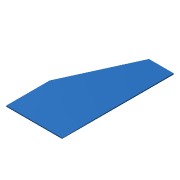
# Autodesk Inventor part: SidePanel
Saved by Autodesk Inventor 2014 (Build 180170000, 170)
## iProperties
Created: 2014-08-10
Part Number: SidePanel
Material: Generic
Document SubType Name: Modeling
Designer: Peele
Density: 1 g/cm^3
Appearance: Cyan
Author: Peele
Autodesk Inventor part; units mm, degrees
ref_plane "YZ Plane" through (0, 0, 0) normal (1, 0, 0) x (0, 1, 0)
ref_plane "XZ Plane" through (0, 0, 0) normal (0, 1, 0) x (-1, 0, 0)
ref_plane "XY Plane" through (0, 0, 0) normal (0, 0, 1) x (1, 0, 0)
sketch "Sketch1" plane through (0, 0, 0) normal (0, 0, 1) x (1, 0, 0)
  line L0 (-112.5, -225) -> (112.5, -225)
  line L1 (112.5, -225) -> (112.5, 225)
  line L2 (112.5, 225) -> (-112.5, 225)
  line L3 (-112.5, 225) -> (-112.5, -225)
  line L4 (-112.5, -225) -> (112.5, 225) construction
  line L5 (112.5, -225) -> (-112.5, 225) construction
  point P0 (0, 0)
  dimension "d0" = 225
  dimension "d1" = 450
  constraints: 12 end point, 2 midpoint, 2 parallel, 1 horizontal, 1 perpendicular
  measures "d0" distance of L1.end L2.end
  measures "d1" distance of L2.end L0.start
extrude "Extrusion1" add sketch "Sketch1" along normal blind 4
sketch "Sketch2" plane through (0, 0, 4) normal (0, 0, 1) x (1, 0, 0)
  line L0 (-112.5, 225) -> (12.5, 225)
  line L1 (12.5, 225) -> (-112.5, -50)
  line L2 (-112.5, 225) -> (-112.5, -50)
  line L3 (112.5, -225) -> (112.5, 225) projected
  line L4 (112.5, -50) -> (112.5, 225)
  line L5 (112.5, 225) -> (62.5, 225)
  line L6 (-112.5, -225) -> (112.5, -225) projected
  line L7 (-112.5, -50) -> (-112.5, 225)
  line L8 (-112.5, 225) -> (12.5, 225)
  point P0 (0, 0)
  dimension "d8" = 175
  constraints: 14 end point, 3 perpendicular, 1 collinear, 1 horizontal alignment, 1 point on line
  measures "d8" distance from line of L1.end L6
extrude "Extrusion2" cut sketch "Sketch2" against normal blind 4
body "Solid1"
